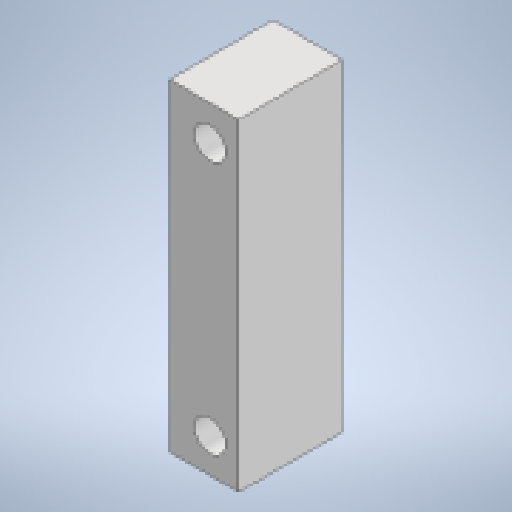
# Autodesk Inventor part: afsd
Saved by Autodesk Inventor 2024 (Build 280153000, 153)
## iProperties
Created: 2024-09-06
Part Number: afsd
Material: PMMA 플라스틱
Document SubType Name: Modeling
Designer: Eungang
Density: 1.188 g/cm^3
Appearance: 폴리카보네이트 - 선명
Author: Eungang
Autodesk Inventor part; units mm, degrees
ref_plane "YZ Plane" through (0, 0, 0) normal (1, 0, 0) x (0, 1, 0)
ref_plane "XZ Plane" through (0, 0, 0) normal (0, 1, 0) x (-1, 0, 0)
ref_plane "XY Plane" through (0, 0, 0) normal (0, 0, 1) x (1, 0, 0)
sketch "스케치1" plane through (0, 0, 0) normal (0, 0, 1) x (1, 0, 0)
  line L0 (-22.85, 14) -> (53.375, 14) projected
  arc A0 (-22.85, 14) -> (-34.1366, 8.2833) centre (-22.85, 0) ccw projected
  arc A1 (-34.1366, 8.2833) -> (-32.5242, 5.1) centre (-32.5242, 7.1) ccw projected
  line L1 (-22.85, 5.1) -> (-32.5242, 5.1) projected
  arc A2 (-22.85, -5.1) -> (-22.85, 5.1) centre (-22.85, 0) ccw projected
  line L2 (-32.5242, -5.1) -> (-22.85, -5.1) projected
  arc A3 (-32.5242, -5.1) -> (-34.1366, -8.2833) centre (-32.5242, -7.1) ccw projected
  arc A4 (-34.1366, -8.2833) -> (-22.85, -14) centre (-22.85, 0) ccw projected
  line L3 (53.375, -14) -> (-22.85, -14) projected
  line L4 (53.375, 14) -> (53.375, -14) projected
  circle A5 centre (-15.0718, 7.7782) radius 1.025 projected
  circle A6 centre (-15.0718, -7.7782) radius 1.025 projected
  circle A7 centre (-22.85, -11) radius 1.025 projected
  circle A8 centre (-22.85, 11) radius 1.025 projected
  circle A9 centre (-30.6282, -7.7782) radius 1.025 projected
  circle A10 centre (-11.85, 0) radius 1.025 projected
  circle A11 centre (-30.6282, 7.7782) radius 1.025 projected
  circle A12 centre (50.8741, 11) radius 1.35 projected
  circle A13 centre (50.8741, -11) radius 1.35 projected
  line L5 (53.375, 14) -> (47.375, 14)
  line L6 (47.375, 14) -> (47.375, -14)
  line L7 (47.375, -14) -> (53.375, -14)
  line L8 (53.375, -14) -> (53.375, 14)
  point P0 (0, 0)
  dimension "d0" = 6
  constraints: 8 end point, 2 parallel, 1 horizontal, 1 perpendicular, 1 point on line
  measures "d0" distance of L7.end L6.end
extrude "돌출1" add sketch "스케치1" along normal blind 8.8 contours L0 L4 L3 L6
sketch "스케치2" plane through (47.375, -14, 0) normal (-1, 0, 0) x (0, 0, 1)
  line L0 (0, 14) -> (0, 11)
  line L1 (0, 28) -> (0, 0) projected
  line L2 (-6.2, 17.1) -> (-6.2, 28) projected
  line L3 (-6.2, 28) -> (0, 28) projected
  line L4 (-0.2, 17.1) -> (-0.2, 28) projected
  line L5 (0, 11) -> (-6.2, 11)
  line L6 (-6.2, 11) -> (-6.2, 17)
  line L7 (-6.2, 17) -> (0, 17)
  line L8 (0, 17) -> (0, 11)
  line L9 (-0.2, 17.1) -> (-6.2, 17.1) projected
  point P0 (-6, 11)
  point P1 (0, 17.1)
  dimension "d3" = 3
  constraints: 10 end point, 2 parallel, 2 point on line, 1 horizontal, 1 perpendicular, 1 other
  measures "d3" distance of L0.start L0.end
extrude "돌출2" add sketch "스케치2" against normal blind 6 contours L0 L5 L6 L7 L1
